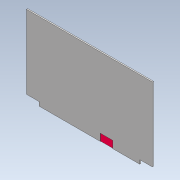
# Autodesk Inventor part: Матрица от ноутбука 15.6 NV156FHM-N42ipt
Saved by Autodesk Inventor 2021.2 (Build 252289000, 289)
## iProperties
Created: 2022-11-28
Part Number: Матрица от ноутбука 15.6 NV156FHM-N42ipt
Material: Типовые
Document SubType Name: Modeling
Designer: Voodoo
Mass: 252.6 g
Surface Area: 1542.11 cm^2
Volume: 252.6 cm^3
Density: 1 g/cm^3
Appearance: По умолчанию
Author: Voodoo
Autodesk Inventor part; units mm, degrees
ref_plane "YZ Plane" through (0, 0, 0) normal (1, 0, 0) x (0, 1, 0)
ref_plane "XZ Plane" through (0, 0, 0) normal (0, 1, 0) x (-1, 0, 0)
ref_plane "XY Plane" through (0, 0, 0) normal (0, 0, 1) x (1, 0, 0)
sketch "Эскиз1" plane through (0, 0, 0) normal (0, 0, 1) x (1, 0, 0)
  line L0 (0, 0) -> (350.66, 0)
  line L1 (350.66, 0) -> (350.66, 205.25)
  line L2 (350.66, 205.25) -> (0, 205.25)
  line L3 (0, 205.25) -> (0, 0)
  line L4 (3.25, 202) -> (347.41, 202)
  line L5 (347.41, 202) -> (347.41, 8.5)
  line L6 (347.41, 8.5) -> (3.25, 8.5)
  line L7 (3.25, 8.5) -> (3.25, 202)
  line L8 (35.18, 0) -> (315.48, 0)
  line L9 (315.48, 0) -> (315.48, -11)
  line L10 (315.48, -11) -> (35.18, -11)
  line L11 (35.18, -11) -> (35.18, 0)
  line L12 (175.33, 8.5) -> (175.33, 37.7602)
  point P0 (175.33, 202)
  point P1 (175.33, 205.25)
  point P2 (175.33, -11)
  dimension "d0" = 350.66
  dimension "d1" = 205.25
  dimension "d2" = 344.16
  dimension "d3" = 193.5
  dimension "d4" = 3.25
  dimension "d5" = 8.5
  dimension "d6" = 3.25
  dimension "d7" = 216.25
  dimension "d9" = 280.3
  dimension "d28" = 35.18
  constraints: 26 end point, 6 parallel, 4 midpoint, 3 horizontal, 3 perpendicular, 2 vertical alignment, 1 point on line, 1 vertical
  measures "d0" distance of L1.end L2.end
  measures "d1" distance of L2.end L0.start
  measures "d2" distance of L4.start L4.end
  measures "d3" distance of L6.end L4.start
  measures "d4" distance between parallel lines of L2 L4
  measures "d5" distance between parallel lines of L6 L0
  measures "d6" distance between parallel lines of L7 L3
  measures "d7" distance between parallel lines of L2 L10
  measures "d9" distance of L9.end L10.end
  measures "d28" distance between parallel lines of L9 L1
extrude "Выдавливание1" add sketch "Эскиз1" along normal blind 3.2
sketch "Эскиз2" plane through (0, 0, 3.2) normal (0, 0, 1) x (1, 0, 0)
  line L0 (0, 0) -> (35.18, 0) projected
  line L1 (35.18, 0) -> (35.18, -11) projected
  line L2 (35.18, -11) -> (315.48, -11) projected
  line L3 (315.48, -11) -> (315.48, 0) projected
  line L4 (315.48, 0) -> (350.66, 0) projected
  line L5 (350.66, 0) -> (350.66, 205.25) projected
  line L6 (350.66, 205.25) -> (0, 205.25) projected
  line L7 (0, 205.25) -> (0, 0) projected
  line L8 (347.41, 202) -> (347.41, 8.5) projected
  line L9 (347.41, 8.5) -> (3.25, 8.5) projected
  line L10 (3.25, 8.5) -> (3.25, 202) projected
  line L11 (3.25, 202) -> (347.41, 202) projected
extrude "Выдавливание2" add sketch "Эскиз2" against normal blind 3.4 contours L8 L9 L10 L11
sketch "Эскиз3" plane through (0, 0, 0) normal (0, 0, -1) x (-1, 0, 0)
  line L0 (0, 0) -> (-35.18, 0) projected
  line L1 (0, 205.25) -> (0, 0) projected
  line L2 (-350.66, 205.25) -> (0, 205.25) projected
  line L3 (-350.66, 0) -> (-350.66, 205.25) projected
  line L4 (-315.48, 0) -> (-350.66, 0) projected
  line L5 (-315.48, -11) -> (-315.48, 0) projected
  line L6 (-35.18, -11) -> (-315.48, -11) projected
  line L7 (-35.18, 0) -> (-35.18, -11) projected
  line L8 (-347.41, 202) -> (-347.41, 8.5) projected
  line L9 (-3.25, 202) -> (-347.41, 202) projected
  line L10 (-3.25, 8.5) -> (-3.25, 202) projected
  line L11 (-347.41, 8.5) -> (-3.25, 8.5) projected
  line L12 (-175.33, -11) -> (-175.33, 1.1845)
  line L13 (-235.57, 5.5) -> (-210.63, 5.5)
  line L14 (-210.63, 5.5) -> (-210.63, 3.5)
  line L15 (-210.63, 3.5) -> (-235.57, 3.5)
  line L16 (-235.57, 3.5) -> (-235.57, 5.5)
  line L17 (-319.31, 5.5) -> (-294.37, 5.5)
  line L18 (-294.37, 5.5) -> (-294.37, 3.5)
  line L19 (-294.37, 3.5) -> (-319.31, 3.5)
  line L20 (-319.31, 3.5) -> (-319.31, 5.5)
  line L21 (-115.09, 5.5) -> (-140.03, 5.5)
  line L22 (-140.03, 5.5) -> (-140.03, 3.5)
  line L23 (-140.03, 3.5) -> (-115.09, 3.5)
  line L24 (-115.09, 3.5) -> (-115.09, 5.5)
  line L25 (-31.35, 5.5) -> (-56.29, 5.5)
  line L26 (-56.29, 5.5) -> (-56.29, 3.5)
  line L27 (-56.29, 3.5) -> (-31.35, 3.5)
  line L28 (-31.35, 3.5) -> (-31.35, 5.5)
  point P0 (-294.37, 4.5)
  point P1 (-235.57, 4.5)
  point P2 (-56.29, 4.5)
  point P3 (-115.09, 4.5)
  dimension "d14" = 24.94
  dimension "d15" = 35.3
  dimension "d16" = 3
  dimension "d17" = 2
  dimension "d18" = 2
  dimension "d19" = 24.94
  dimension "d20" = 58.8
  constraints: 34 end point, 10 symmetric about line, 4 parallel, 4 point on line, 3 midpoint, 2 horizontal, 2 perpendicular, 1 horizontal alignment, 1 vertical
  measures "d14" distance of L14.end L15.end
  measures "d15" distance from line of L14.end L12
  measures "d16" distance between parallel lines of L11 L13
  measures "d17" distance of L13.end L14.end
  measures "d18" distance between parallel lines of L17 L19
  measures "d19" distance of L18.end L19.end
  measures "d20" distance of point (-235.57, 4.5) point (-294.37, 4.5)
extrude "Выдавливание3" cut sketch "Эскиз3" against normal blind 1 contours L13 L14 L15 L16 | L17 L18 L19 L20 | L24 L23 L22 L21 | L28 L27 L26 L25
sketch "Эскиз5" plane through (0, 0, 3.2) normal (0, 0, 1) x (1, 0, 0)
  line L0 (0, 0) -> (35.18, 0) projected
  line L1 (35.18, 0) -> (35.18, -11) projected
  line L2 (35.18, -11) -> (315.48, -11) projected
  line L3 (315.48, -11) -> (315.48, 0) projected
  line L4 (315.48, 0) -> (350.66, 0) projected
  line L5 (350.66, 0) -> (350.66, 205.25) projected
  line L6 (350.66, 205.25) -> (0, 205.25) projected
  line L7 (0, 205.25) -> (0, 0) projected
  line L8 (205.66, -11) -> (240.66, -11)
  line L9 (240.66, -11) -> (240.66, 9)
  line L10 (240.66, 9) -> (205.66, 9)
  line L11 (205.66, 9) -> (205.66, -11)
  dimension "d23" = 110
  dimension "d24" = 20
  dimension "d25" = 35
  constraints: 8 end point, 2 parallel, 1 collinear, 1 horizontal, 1 perpendicular
  measures "d23" distance between parallel lines of L5 L9
  measures "d24" distance of L8.end L9.end
  measures "d25" distance of L9.end L10.end
extrude "Выдавливание4" cut sketch "Эскиз5" against normal blind 1 contours L11 L10 L9 L2
equation "\"d19\" = d14"
